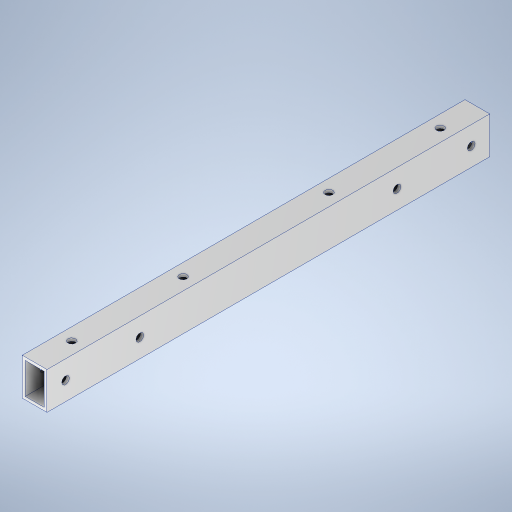
# Autodesk Inventor part: base_pipe1
Saved by Autodesk Inventor 2024 (Build 280153000, 153)
## iProperties
Created: 2025-02-13
Part Number: base_pipe1
Material: アルミニウム 6061
Document SubType Name: Modeling
Designer: tanoue_kota
Density: 2.7 g/cm^3
Appearance: アルミニウム - フラット
Author: tanoue_kota
Autodesk Inventor part; units mm, degrees
ref_plane "YZ Plane" through (0, 0, 0) normal (1, 0, 0) x (0, 1, 0)
ref_plane "XZ Plane" through (0, 0, 0) normal (0, 1, 0) x (-1, 0, 0)
ref_plane "XY Plane" through (0, 0, 0) normal (0, 0, 1) x (1, 0, 0)
sketch "スケッチ1" plane through (0, 0, 0) normal (0, 1, 0) x (-1, 0, 0)
  line L0 (0, 0) -> (10, 0)
  line L1 (10, 0) -> (10, 178.952)
  line L2 (10, 178.952) -> (0, 178.952)
  line L3 (0, 178.952) -> (0, 0)
  dimension "d0" = 10
  dimension "d1" = 178.952
  constraints: 8 end point, 2 parallel, 1 horizontal, 1 perpendicular
  measures "d0" distance of L1.end L2.end
  measures "d1" distance of L0.end L1.end
extrude "押し出し1" add sketch "スケッチ1" along normal blind 15
shell "シェル1" thickness 1.2 removed faces 2 at (-3.3333, 5, 0) at (-6.6667, 5, 178.952)
sketch "スケッチ2" plane through (-10, 0, 0) normal (-1, 0, 0) x (0, 0, 1)
  line L0 (0, 1.2) -> (0, 13.8) projected
  line L1 (0, 7.5) -> (178.952, 7.5)
  line L2 (178.952, 1.2) -> (178.952, 13.8) projected
  point P0 (0, 0)
  point P1 (171.452, 7.5)
  point P2 (141.452, 7.5)
  point P3 (7.5, 7.5)
  point P4 (37.5, 7.5)
  dimension "d5" = 7.5
  dimension "d6" = 30
  dimension "d7" = 7.5
  dimension "d8" = 30
  constraints: 4 point on line, 2 end point, 2 midpoint
  measures "d5" distance from line of L2 point (171.452, 7.5)
  measures "d6" distance of point (171.452, 7.5) point (141.452, 7.5)
  measures "d7" distance from line of L0 point (7.5, 7.5)
  measures "d8" distance of point (7.5, 7.5) point (37.5, 7.5)
hole "穴1" at (-10, 7.5, 171.452) at (-10, 7.5, 141.452) at (-10, 7.5, 7.5) at (-10, 7.5, 37.5) direction (1, 0, 0) diameter 3.1 end through all
sketch "スケッチ3" plane through (0, 15, 0) normal (0, 1, 0) x (1, 0, 0)
  line L0 (0, 0) -> (-10, 0) projected
  line L1 (-5, 0) -> (-5, -178.952)
  line L2 (-10, -178.952) -> (0, -178.952) projected
  point P0 (-5, -15)
  point P1 (-5, -60)
  point P2 (-5, -163.952)
  point P3 (-5, -118.952)
  dimension "d16" = 15
  dimension "d17" = 45
  dimension "d18" = 15
  dimension "d19" = 45
  constraints: 4 point on line, 2 end point, 2 midpoint
  measures "d16" distance from line of L0 point (-5, -15)
  measures "d17" distance of point (-5, -15) point (-5, -60)
  measures "d18" distance from line of L2 point (-5, -163.952)
  measures "d19" distance of point (-5, -163.952) point (-5, -118.952)
hole "穴2" at (-5, 15, 15) at (-5, 15, 60) at (-5, 15, 163.952) at (-5, 15, 118.952) direction (0, -1, 0) diameter 3.1 end through all
sketch "スケッチ4" plane through (0, 15, 0) normal (0, 1, 0) x (1, 0, 0)
  circle A0 centre (-5, -118.952) radius 1.55 projected
  circle A1 centre (-5, -60) radius 1.55 projected
  line L0 (-5, -118.952) -> (-5, -60)
  line L1 (-5, -89.476) -> (-135, -89.476)
  circle A2 centre (-70, -90.476) radius 88
  line L2 (-70, -90.476) -> (-7.7746, -28.2506)
  line L3 (-5, -90.476) -> (-135, -90.476)
  point P0 (0, 0)
  point P1 (-132.2254, -28.2506)
  point P2 (-132.2254, -152.7014)
  point P3 (-7.7746, -152.7014)
  dimension "d30" = 176
  dimension "d27" = 130
  dimension "d34" = 360
  dimension "d47" = 1
  constraints: 8 end point, 4 coincident, 2 midpoint, 1 horizontal, 1 parallel, 1 vertical, 8 other
  measures "d27" distance of L1.start L1.end
  measures "d47" distance between parallel lines of L1 L3
hole "穴3" [suppressed]
